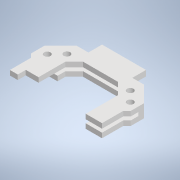
# Autodesk Inventor part: Button Holder
Saved by Autodesk Inventor 2020 (Build 240168000, 168)
## iProperties
Created: 2021-01-14
Part Number: Button Holder
Material: Generic
Document SubType Name: Modeling
Designer: Luke
Density: 1 g/cm^3
Appearance: Default
Author: Luke
Autodesk Inventor part; units mm, degrees
ref_plane "YZ Plane" through (0, 0, 0) normal (1, 0, 0) x (0, 1, 0)
ref_plane "XZ Plane" through (0, 0, 0) normal (0, 1, 0) x (-1, 0, 0)
ref_plane "XY Plane" through (0, 0, 0) normal (0, 0, 1) x (1, 0, 0)
ref_plane "Work Plane1" through (59.9208, 47.0911, 21.911) normal (0, 1, 0) x (-1, 0, 0)
sketch "Sketch1" plane through (59.9208, 47.0911, 21.911) normal (0, 1, 0) x (-1, 0, 0)
  circle A0 centre (-16.808, -43.6345) radius 1.27
  circle A1 centre (12.5729, -47.6345) radius 1.27
  circle A2 centre (16.4459, -43.6345) radius 1.27
  circle A3 centre (-12.808, -47.6345) radius 1.27
  line L0 (10.208, -33.8805) -> (10.208, -44.6601)
  line L1 (10.208, -44.6601) -> (6.6725, -48.1956)
  circle A4 centre (-16.808, -43.6345) radius 1.27 projected
  circle A5 centre (12.5729, -47.6345) radius 1.27 projected
  circle A6 centre (16.4459, -43.6345) radius 1.27 projected
  circle A7 centre (-12.8081, -47.6345) radius 1.27 projected
  line L2 (19.708, -15.6655) -> (-19.708, -15.6655)
  line L3 (0, -15.6655) -> (0, -20.8781)
  line L4 (6.6725, -48.1956) -> (-7.3796, -48.1956)
  line L5 (-19.958, -43.8381) -> (-12.8316, -50.9645)
  line L6 (-12.8316, -50.9645) -> (12.8316, -50.9645)
  line L7 (-19.958, -40.6601) -> (-19.958, -43.8381)
  line L8 (0, -48.1956) -> (0, -46.7038)
  line L9 (19.958, -43.8381) -> (12.8316, -50.9645)
  line L10 (19.958, -40.6601) -> (19.958, -43.8381)
  line L11 (-11.938, -30.6601) -> (-11.938, -43.6372)
  line L12 (-10.5616, -45.0137) -> (-11.938, -43.6372)
  line L13 (-10.5616, -45.0137) -> (-7.3796, -48.1956)
  line L14 (15.2967, -30.6601) -> (18.458, -30.6601)
  line L15 (18.458, -30.6601) -> (18.458, -39.1601)
  line L16 (-18.458, -39.1601) -> (-18.458, -30.6601)
  line L17 (-18.458, -30.6601) -> (-11.938, -30.6601)
  line L18 (10.208, -33.8805) -> (15.2967, -33.8805)
  line L19 (15.2967, -33.8805) -> (15.2967, -30.6601)
  line L20 (-19.958, -40.6601) -> (-18.458, -39.1601)
  line L21 (19.958, -40.6601) -> (18.458, -39.1601)
  point P0 (-19.708, -43.6601)
  point P1 (-6.6725, -48.1956)
  dimension "d14" = 5
  dimension "d15" = 135
  dimension "d18" = 2.54
  constraints: 44 end point, 4 centre point, 4 symmetric about line, 3 vertical, 2 horizontal, 2 point on line, 1 midpoint, 1 perpendicular
  measures "d14" distance of L0.end L1.end
  measures "d15" angle of L0 L1
  measures "d18" diameter of A1
extrude "Extrusion1" add sketch "Sketch1" along normal blind 2
ref_plane "Work Plane2" through (59.9208, 45.8611, 21.911) normal (0, -1, 0) x (1, 0, 0)
sketch "Sketch2" plane through (59.9208, 45.8611, 21.911) normal (0, -1, 0) x (1, 0, 0)
  line L0 (-10.208, -33.8805) -> (-10.208, -44.6601) projected
  line L1 (-10.208, -44.6601) -> (-6.6725, -48.1956) projected
  line L2 (-6.6725, -48.1956) -> (7.3796, -48.1956) projected
  circle A0 centre (16.808, -43.6345) radius 1.27 projected
  circle A1 centre (-12.5729, -47.6345) radius 1.27 projected
  circle A2 centre (-16.4459, -43.6345) radius 1.27 projected
  circle A3 centre (12.808, -47.6345) radius 1.27 projected
  line L3 (19.958, -40.6601) -> (19.958, -43.8381) projected
  line L4 (19.958, -43.8381) -> (12.8316, -50.9645) projected
  line L5 (12.8316, -50.9645) -> (-12.8316, -50.9645) projected
  line L6 (-12.8316, -50.9645) -> (-19.958, -43.8381) projected
  line L7 (-19.958, -43.8381) -> (-19.958, -40.6601) projected
  line L8 (7.3796, -48.1956) -> (11.938, -43.6372) projected
  line L9 (11.938, -43.6372) -> (11.938, -30.6601) projected
  line L10 (11.938, -30.6601) -> (18.458, -30.6601) projected
  line L11 (18.458, -30.6601) -> (18.458, -39.1601) projected
  line L12 (-18.458, -39.1601) -> (-18.458, -30.6601) projected
  line L13 (-18.458, -30.6601) -> (-15.2967, -30.6601) projected
  line L14 (-15.2967, -30.6601) -> (-15.2967, -33.8805) projected
  line L15 (-15.2967, -33.8805) -> (-10.208, -33.8805) projected
  line L16 (18.458, -39.1601) -> (19.958, -40.6601) projected
  line L17 (-19.958, -40.6601) -> (-18.458, -39.1601) projected
  circle A4 centre (-16.4459, -43.6345) radius 1.27 projected
  line L18 (-19.958, -43.8381) -> (-19.958, -40.6601) projected
  line L19 (-19.958, -41.5123) -> (-10.208, -41.5123)
  line L20 (-10.208, -33.8805) -> (-10.208, -44.6601) projected
  point P0 (-59.9208, -21.911)
  constraints: 2 end point, 1 perpendicular, 1 point on line
extrude "Extrusion2" add sketch "Sketch2" along normal blind 2 contours L0 L1 L2 L8 L9 L10 L11 L16 L3 L4 L5 L6 L7 L19
sketch "Sketch4" plane through (79.8789, 45.8611, -18.7491) normal (1, 0, 0) x (0, 0, -1)
  line L0 (0, 1.23) -> (3.178, 1.23) projected
  line L1 (0, 0) -> (-1.5, 0) projected
  line L2 (0, 1.23) -> (0, 0)
  line L3 (-12.1065, -0.085) -> (12.1065, -0.085)
  line L4 (12.1065, -0.085) -> (12.1065, 1.315)
  line L5 (12.1065, 1.315) -> (-12.1065, 1.315)
  line L6 (-12.1065, 1.315) -> (-12.1065, -0.085)
  line L7 (-12.1065, -0.085) -> (12.1065, 1.315) construction
  line L8 (12.1065, -0.085) -> (-12.1065, 1.315) construction
  point P0 (0, 0.615)
  dimension "d73" = 1.4
  constraints: 14 end point, 3 midpoint, 2 parallel, 1 horizontal, 1 perpendicular, 1 vertical
  measures "d73" distance of L4.end L3.end
extrude "Extrusion3" cut sketch "Sketch4" against normal through all
sketch "Sketch5" plane through (59.9208, 43.8611, 21.911) normal (0, -1, 0) x (1, 0, 0)
  line L0 (-19.708, -43.6601) -> (-19.708, -40.6601)
  line L1 (-12.6424, -50.7145) -> (-19.708, -43.6601)
  line L2 (12.728, -50.7145) -> (-12.6424, -50.7145)
  line L3 (19.708, -43.7345) -> (12.728, -50.7145)
  line L4 (-13.4529, -52.4645) -> (13.4529, -52.4645)
  line L5 (19.708, -43.7345) -> (19.708, -40.6601)
  line L6 (-12.8316, -50.9145) -> (12.8316, -50.9145)
  line L7 (12.8316, -50.9645) -> (11.3316, -52.4645)
  line L8 (-19.958, -43.8381) -> (-12.8316, -50.9645)
  line L9 (-12.8316, -50.9645) -> (-11.3316, -52.4645)
  line L10 (-12.8316, -50.9645) -> (-10.7103, -50.9645) construction
  line L11 (12.8316, -50.9145) -> (12.8816, -50.9145)
  line L12 (-12.8316, -50.9645) -> (12.8316, -50.9645)
  line L13 (12.8316, -50.9645) -> (12.8816, -50.9145)
  line L14 (12.8316, -50.9645) -> (19.958, -43.8381)
  line L15 (-12.8316, -50.9145) -> (-12.8816, -50.9145)
  line L16 (-12.8316, -50.9645) -> (-12.8816, -50.9145)
  line L17 (12.8109, -50.9145) -> (19.958, -43.7673)
  line L18 (-19.958, -43.7673) -> (-12.8109, -50.9145)
  line L19 (-19.958, -45.9594) -> (-13.4529, -52.4645)
  line L20 (13.4529, -52.4645) -> (19.958, -45.9594)
  line L21 (-19.958, -43.7673) -> (-19.958, -45.9594)
  line L22 (12.8316, -50.9645) -> (19.958, -43.8381) projected
  line L23 (19.958, -43.8381) -> (19.958, -45.9594)
  line L24 (19.958, -43.8381) -> (19.958, -43.7673)
  line L25 (19.958, -43.8381) -> (19.958, -40.6601) projected
  dimension "d29" = 0.2
  dimension "d62" = 45
  dimension "d74" = 0.05
  dimension "d75" = 0.05
  dimension "d76" = 1.5
  dimension "d77" = 1.5
  constraints: 48 end point, 7 point on line, 4 parallel, 3 horizontal, 2 vertical, 1 equal length
  measures "d29" distance between parallel lines of L2 L6
  measures "d62" angle of L9 L10
  measures "d74" distance between parallel lines of L14 L17
  measures "d75" distance between parallel lines of L8 L18
  measures "d76" distance between parallel lines of L8 L19
  measures "d77" distance between parallel lines of L14 L20
extrude "Extrusion4" add sketch "Sketch5" against normal up to surface (5.23 mm away)
ref_plane "Work Plane13" through (59.9208, 43.8611, -18.7491) normal (1, 0, 0) x (0, 0, -1)
ref_plane "Work Plane14" through (53.2483, 46.4761, -26.2847) normal (0, 1, 0) x (1, 0, 0)
sketch "Sketch18" plane through (59.9208, 43.8611, -18.7491) normal (1, 0, 0) x (0, 0, -1)
  line L0 (11.8044, -3.849) -> (14.1534, -3.849)
  line L1 (14.1534, -3.849) -> (15.5534, -3.849)
  line L2 (15.5534, -3.849) -> (15.5534, -2.0485)
  line L3 (15.5534, -2.0485) -> (14.3033, -2.0485)
  line L4 (14.3033, -2.0485) -> (14.3033, 0.7794)
  line L5 (14.3033, 0.7794) -> (13.0544, 0.7794)
  line L6 (13.0544, 0.7794) -> (13.0544, 2.98)
  line L7 (13.0544, 2.98) -> (14.6544, 2.98)
  line L8 (14.6544, 2.98) -> (17.2804, 2.98)
  line L9 (17.2804, 2.98) -> (17.2804, 5.23)
  line L10 (17.2804, 5.23) -> (13.0544, 5.23)
  line L11 (13.0544, 5.23) -> (11.8044, 5.23)
  line L12 (5.2993, 5.23) -> (11.8044, 5.23) projected
  line L13 (11.8044, 0) -> (11.8044, 5.23) projected
  line L14 (11.8044, 5.23) -> (11.8044, -3.849)
  dimension "d164" = 1.25
  dimension "d165" = 180
  dimension "d176" = 90
  constraints: 26 end point, 4 perpendicular, 1 vertical
  measures "d164" distance of L10.end L11.end
  measures "d165" angle of L10 L11
  measures "d176" angle of L4 L5
extrude "Extrusion12" add sketch "Sketch18" along normal blind 8.804 and the other way blind 8.804
chamfer "Chamfer7" distance 1.5 angle 45 1 edges at (59.9208, 43.8611, -30.5535)
ref_plane "Work Plane17" through (51.1168, 46.6411, -36.0296) normal (0, -1, 0) x (1, 0, 0)
ref_plane "Work Plane18" through (68.7248, 44.6406, -33.2524) normal (0, 0, -1) x (-1, 0, 0)
body "Solid1"
